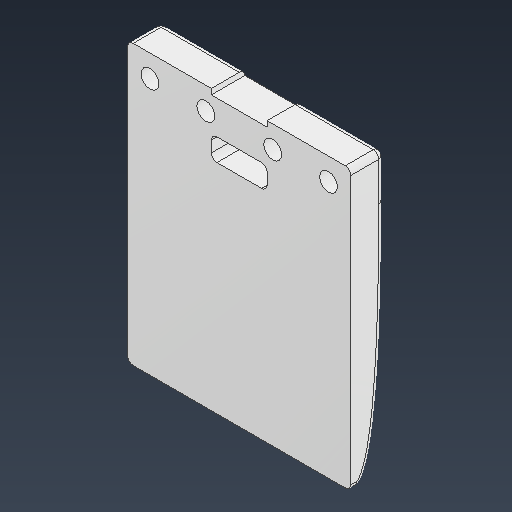
# Autodesk Inventor part: base22
Saved by Autodesk Inventor 2021 (Build 250183000, 183)
## iProperties
Created: 2021-08-08
Part Number: base22
Material: ABS プラスチック
Document SubType Name: Modeling
Designer: yuta0
Density: 1.06 g/cm^3
Appearance: 滑らか - 白
Mass: 10.6859 g
Surface Area: 50.4158 cm^2
Volume: 10.0811 cm^3
在庫数: 0.0
購入先: 印刷
Author: yuta0
Autodesk Inventor part; units mm, degrees
ref_plane "YZ Plane" through (0, 0, 0) normal (1, 0, 0) x (0, 1, 0)
ref_plane "XZ Plane" through (0, 0, 0) normal (0, 1, 0) x (-1, 0, 0)
ref_plane "XY Plane" through (0, 0, 0) normal (0, 0, 1) x (1, 0, 0)
sketch "スケッチ3" plane through (0, 0, 0) normal (1, 0, 0) x (0, 1, 0)
  line L0 (0, 0) -> (50, 0)
  line L1 (50, 0) -> (50, -6)
  line L2 (50, -6) -> (42, -6)
  line L3 (0, 0) -> (0, -1)
  line L4 (0, -1) -> (0, -6) construction
  line L5 (0, -6) -> (42, -6) construction
  spline S0 degree 2 poles (0, -1) (0, -6) (42, -6) knots 1 1 1 2 2 2
  dimension "d14" = 6
  dimension "d15" = 1
  dimension "d16" = 8
  dimension "d17" = 50
  constraints: 8 end point, 3 perpendicular, 2 vertical, 1 horizontal, 3 other
  measures "d14" distance of L0.end L1.end
  measures "d15" distance of L0.start L3.end
  measures "d16" distance of L1.end L2.end
  measures "d17" distance of L0.start L0.end
extrude "押し出し2" add sketch "スケッチ3" along normal mid plane 40
sketch "スケッチ4" plane through (20, 50, -6) normal (0, 0, -1) x (-1, 0, 0)
  line L0 (0, -8) -> (0, 0) projected
  line L1 (40, 0) -> (0, 0) projected
  point P0 (20, -50)
  point P1 (14, -4)
  point P2 (14, -4)
  point P3 (4, -4)
  dimension "d20" = 4
  dimension "d21" = 4
  dimension "d22" = 10
  constraints: 1 coincident, 1 horizontal alignment
  measures "d20" distance from line of L0 point (4, -4)
  measures "d21" distance from line of L1 point (4, -4)
  measures "d22" distance of point (14, -4) point (4, -4)
hole "穴2" at (6, 46, -6) at (16, 46, -6) direction (0, 0, 1) diameter 3.2 end through all clearance for "Flat Head Machine Screw" size "M3" standard "Ansi Metric M Profile"
fillet "フィレット1" radius 1 9 edges at (20, 10.5, -4.75) (20, 46, -6) (20, 0, -0.5) (-20, 0, -0.5) (-20, 46, -6) (-20, 10.5, -4.75) (0, 50, -6) (-20, 50, -3) (20, 50, -3)
mirror "ミラー1" about plane through (0, 0, 0) normal (1, 0, 0) of "穴2"
sketch "スケッチ5" plane through (-19, 50, 0) normal (0, 0, 1) x (1, 0, 0)
  line L0 (0, -11) -> (38, -11)
  line L1 (38, -11) -> (38, -49)
  line L2 (38, -49) -> (0, -49)
  line L3 (0, -49) -> (0, -11)
  line L4 (0, -11) -> (38, -49) construction
  line L5 (38, -11) -> (0, -49) construction
  line L6 (-1, -49) -> (-1, -1) projected
  line L7 (0, -50) -> (38, -50) projected
  line L8 (14, -11) -> (24, -11)
  line L9 (24, -11) -> (24, -7)
  line L10 (24, -7) -> (14, -7)
  line L11 (14, -7) -> (14, -11)
  line L12 (14, -11) -> (24, -7) construction
  line L13 (24, -11) -> (14, -7) construction
  line L14 (24, -1) -> (14, -1)
  line L15 (14, -1) -> (14, 0)
  line L16 (14, 0) -> (24, 0)
  line L17 (24, 0) -> (24, -1)
  line L18 (24, -1) -> (14, 0) construction
  line L19 (14, -1) -> (24, 0) construction
  line L20 (0, 0) -> (38, 0) projected
  point P0 (19, -50)
  point P1 (19, -30)
  point P2 (19, -9)
  point P3 (19, -9)
  point P4 (19, -30)
  point P5 (24, -11)
  point P6 (19, -0.5)
  point P7 (19, -0.5)
  point P8 (19, -9)
  dimension "d31" = 38
  dimension "d32" = 38
  dimension "d33" = 1
  dimension "d34" = 1
  dimension "d35" = 10
  dimension "d36" = 4
  dimension "d40" = 10
  dimension "d41" = 1
  constraints: 36 end point, 10 midpoint, 6 parallel, 3 horizontal, 3 perpendicular, 2 point on line, 2 vertical alignment
  measures "d31" distance of L1.end L2.end
  measures "d32" distance of L0.end L1.end
  measures "d33" distance between parallel lines of L6 L3
  measures "d34" distance between parallel lines of L7 L2
  measures "d35" distance of L10.end L9.end
  measures "d36" distance of L9.end L8.end
  measures "d40" distance of L14.start L14.end
  measures "d41" distance between parallel lines of L16 L14
extrude "押し出し3" cut sketch "スケッチ5" against normal blind 40 contours L11 L10 L9 L0 | L14 L15 L16 L17
fillet "フィレット2" radius 1 4 edges at (-5, 39, -2.9967) (-5, 43, -3) (5, 43, -3) (5, 39, -2.9967)
